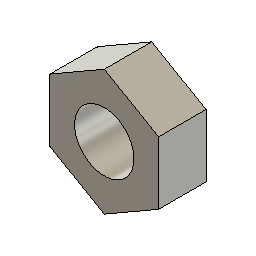
_nut.abc1873e-3841-4139-b8da-671c361234e5 (Autodesk Fusion 360 design; units mm, degrees)
Autodesk Fusion 360 part; units mm, degrees
sketch "Sketch1" plane through (0, 0, 0) normal (0, 0, 1) x (1, 0, 0)
  line L0 (0, 3.175) -> (-2.7496, 1.5875)
  line L1 (-2.7496, 1.5875) -> (-2.7496, -1.5875)
  line L2 (-2.7496, -1.5875) -> (0, -3.175)
  line L3 (0, -3.175) -> (2.7496, -1.5875)
  line L4 (2.7496, -1.5875) -> (2.7496, 1.5875)
  line L5 (2.7496, 1.5875) -> (0, 3.175)
  circle A0 centre (0, 0) radius 1.5
  dimension "d1" = 3.175
  dimension "d2" = 3
  constraint coincident A0.centre origin
  measures "d1" distance of L0.start A0.centre
  measures "d2" diameter of A0
extrude "Extrude1" add sketch "Sketch1" along normal blind 2.4
